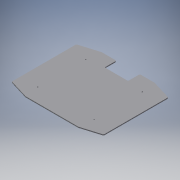
# Autodesk Inventor part: SwarmieCoverPlate
Saved by Autodesk Inventor 2016 (Build 200138000, 138)
## iProperties
Created: 2015-05-25
Part Number: SwarmieCoverPlate
Material: Generic
Document SubType Name: Modeling
Designer: Karl
Density: 1 g/cm^3
Appearance: Default
Author: Karl
Autodesk Inventor part; units mm, degrees
ref_plane "YZ Plane" through (0, 0, 0) normal (1, 0, 0) x (0, 1, 0)
ref_plane "XZ Plane" through (0, 0, 0) normal (0, 1, 0) x (-1, 0, 0)
ref_plane "XY Plane" through (0, 0, 0) normal (0, 0, 1) x (1, 0, 0)
sketch "Sketch1" plane through (0, 0, 0) normal (0, 1, 0) x (-1, 0, 0)
  line L0 (149.225, -123.825) -> (-149.225, -123.825)
  line L1 (-149.225, -123.825) -> (-149.225, 123.825)
  line L2 (-149.225, 123.825) -> (149.225, 123.825)
  line L3 (149.225, 123.825) -> (149.225, -123.825)
  line L4 (149.225, -123.825) -> (-149.225, 123.825) construction
  line L5 (-149.225, -123.825) -> (149.225, 123.825) construction
  point P0 (0, 0)
  dimension "d0" = 298.45
  dimension "d1" = 247.65
  constraints: 12 end point, 2 midpoint, 2 parallel, 1 horizontal, 1 perpendicular
  measures "d0" distance of L1.end L2.end
  measures "d1" distance of L0.end L1.end
extrude "Extrusion1" add sketch "Sketch1" along normal blind 3.175
sketch "Sketch2" plane through (0, 3.175, 0) normal (0, 1, 0) x (1, 0, 0)
  line L0 (149.225, 123.825) -> (-149.225, 123.825) projected
  line L1 (-149.225, 123.825) -> (-149.225, -123.825) projected
  line L2 (-149.225, -123.825) -> (149.225, -123.825) projected
  line L3 (149.225, -123.825) -> (149.225, 123.825) projected
  line L4 (-149.225, 104.775) -> (-85.725, 123.825)
  line L5 (85.725, 123.825) -> (149.225, 104.775)
  line L6 (149.225, -104.775) -> (85.725, -123.825)
  line L7 (-85.725, -123.825) -> (-149.225, -104.775)
  point P0 (0, 0)
  dimension "d4" = 19.05
  dimension "d5" = 19.05
  dimension "d6" = 19.05
  dimension "d7" = 19.05
  dimension "d8" = 63.5
  dimension "d9" = 63.5
  dimension "d10" = 63.5
  constraints: 8 end point, 8 point on line, 1 parallel
  measures "d4" distance from line of L0 L4.start
  measures "d5" distance from line of L2 L7.end
  measures "d6" distance from line of L5.end L0
  measures "d7" distance from line of L2 L6.start
  measures "d8" distance from line of L1 L4.end
  measures "d9" distance from line of L3 L5.start
  measures "d10" distance from line of L1 L7.start
extrude "Extrusion2" cut sketch "Sketch2" against normal blind 3.175 contours L3 L5 L0 | L4 L1 L0 | L3 L2 L6 | L7 L2 L1
sketch "Sketch3" plane through (0, 3.175, 0) normal (0, 1, 0) x (1, 0, 0)
  line L0 (85.725, 123.825) -> (-85.725, 123.825) projected
  line L1 (-38.1, 123.825) -> (38.1, 123.825)
  line L2 (38.1, 123.825) -> (38.1, 85.725)
  line L3 (38.1, 85.725) -> (-38.1, 85.725)
  line L4 (-38.1, 85.725) -> (-38.1, 123.825)
  point P0 (0, 0)
  point P1 (0, 85.725)
  dimension "d13" = 38.1
  dimension "d14" = 76.2
  constraints: 8 end point, 2 parallel, 1 horizontal, 1 midpoint, 1 perpendicular, 1 point on line, 1 vertical alignment
  measures "d13" distance of L3.end L1.start
  measures "d14" distance of L2.end L3.end
extrude "Extrusion3" cut sketch "Sketch3" against normal blind 3.175
fillet "Fillet1" radius 3.175 12 edges at (38.1, 1.5875, -85.725) (-38.1, 1.5875, -85.725) (38.1, 1.5875, -123.825) (-38.1, 1.5875, -123.825) (85.725, 1.5875, -123.825) (-85.725, 1.5875, -123.825) (-149.225, 1.5875, -104.775) (149.225, 1.5875, -104.775) (-149.225, 1.5875, 104.775) (-85.725, 1.5875, 123.825) (85.725, 1.5875, 123.825) (149.225, 1.5875, 104.775)
sketch "Sketch4" plane through (0, 3.175, 0) normal (0, 1, 0) x (1, 0, 0)
  point P0 (0, 0)
  point P1 (-91.6686, 78.105)
  point P2 (-91.6686, -78.105)
  point P3 (91.6686, -78.105)
  point P4 (91.6686, 78.105)
  dimension "d18" = 78.105
  dimension "d19" = 78.105
  dimension "d20" = 91.6686
  dimension "d21" = 91.6686
  constraints: 2 horizontal alignment, 2 vertical alignment
  measures "d18" vertical distance of point (-91.669, -78.105) point (0, 0)
  measures "d19" vertical distance of point (-91.669, 78.105) point (0, 0)
  measures "d20" horizontal distance of point (-91.669, 78.105) point (0, 0)
  measures "d21" horizontal distance of point (91.669, 78.105) point (0, 0)
hole "Hole1" at (-91.6686, 3.175, -78.105) at (-91.6686, 3.175, 78.105) at (91.6686, 3.175, 78.105) at (91.6686, 3.175, -78.105) direction (0, -1, 0) diameter 3.302 end through all
body "Solid1"
